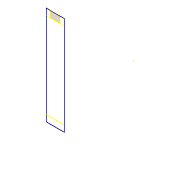
# Autodesk Inventor part: 572000_Bottom Guard
Saved by Autodesk Inventor 2015 (Build 190159000, 159)
## iProperties
Created: 2014-07-17
Part Number: 572000_Bottom Guard
Material: Polycarbonate, Clear
Document SubType Name: Modeling
Designer: david
Density: 1.2 g/cm^3
Appearance: Polycarbonate - Clear
Author: david
Autodesk Inventor part; units mm, degrees
ref_plane "YZ Plane" through (0, 0, 0) normal (1, 0, 0) x (0, 1, 0)
ref_plane "XZ Plane" through (0, 0, 0) normal (0, 1, 0) x (-1, 0, 0)
ref_plane "XY Plane" through (0, 0, 0) normal (0, 0, 1) x (1, 0, 0)
ref_plane "Work Plane4" through (0, 0, 0) normal (0, 0, 1) x (1, 0, 0)
sketch "Sketch1" plane through (0, 0, 0) normal (0, 0, 1) x (1, 0, 0)
  line L0 (-206.1633, -12.7) -> (-206.1633, 6.35) projected
  line L1 (-206.1633, 6.35) -> (-259.9103, 6.35) projected
  line L2 (-259.9103, -12.7) -> (-259.9103, 6.35) projected
  line L3 (-206.1633, -12.7) -> (-259.9103, -12.7) projected
  line L4 (-206.1633, -12.7) -> (-206.1633, 6.35) projected
  line L5 (-259.8883, -285.75) -> (-206.1413, -285.75) projected
  line L6 (-206.1413, -266.7) -> (-206.1413, -285.75) projected
  line L7 (-259.8883, -266.7) -> (-206.1413, -266.7) projected
  line L8 (-259.8883, -266.7) -> (-259.8883, -285.75) projected
  line L9 (-259.9103, 6.35) -> (-206.1413, 6.35)
  line L10 (-206.1413, 6.35) -> (-206.1413, -285.75)
  line L11 (-206.1413, -285.75) -> (-259.9103, -285.75)
  line L12 (-259.9103, -285.75) -> (-259.9103, 6.35)
  point P0 (0, 0)
  constraints: 8 end point, 2 parallel, 1 horizontal, 1 perpendicular
extrude "Extrusion1" add sketch "Sketch1" along normal blind 1.5875
body "Solid1"
